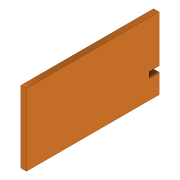
# Autodesk Inventor part: bottom_inner_wall
Saved by Autodesk Inventor 2020 (Build 240168000, 168)
## iProperties
Created: 2021-05-08
Part Number: bottom_inner_wall
Material: Gold
Document SubType Name: Modeling
Designer: Hsu Daniel
Density: 19.3 g/cm^3
Appearance: Metal 1600F Hot
Author: Hsu Daniel
Autodesk Inventor part; units mm, degrees
ref_plane "YZ Plane" through (0, 0, 0) normal (1, 0, 0) x (0, 1, 0)
ref_plane "XZ Plane" through (0, 0, 0) normal (0, 1, 0) x (-1, 0, 0)
ref_plane "XY Plane" through (0, 0, 0) normal (0, 0, 1) x (1, 0, 0)
sketch "Sketch1" plane through (0, 0, 0) normal (1, 0, 0) x (0, 1, 0)
  line L0 (0, 0) -> (71.7, 0)
  line L1 (71.7, 0) -> (71.7, -132.6)
  line L2 (71.7, -132.6) -> (0, -132.6)
  line L3 (0, -132.6) -> (0, 0)
  dimension "d0" = 71.7
  dimension "d1" = 132.6
  constraints: 8 end point, 2 parallel, 1 horizontal, 1 perpendicular
  measures "d0" distance of L1.end L2.end
  measures "d1" distance of L0.end L1.end
extrude "Extrusion1" add sketch "Sketch1" along normal blind 5.5
sketch "Sketch4" plane through (0, 0, 0) normal (-1, 0, 0) x (0, 0, 1)
  line L0 (-132.6, 0) -> (-132.6, 71.7) projected
  line L1 (-132.6, 25) -> (-122.6, 25)
  line L2 (-122.6, 25) -> (-122.6, 19.5)
  line L3 (-122.6, 19.5) -> (-132.6, 19.5)
  line L4 (-132.6, 19.5) -> (-132.6, 25)
  line L5 (0, 0) -> (-132.6, 0) projected
  dimension "d12" = 10
  dimension "d13" = 5.5
  dimension "d14" = 25
  constraints: 8 end point, 2 parallel, 1 horizontal, 1 perpendicular, 1 point on line
  measures "d12" distance of L2.end L3.end
  measures "d13" distance of L1.end L2.end
  measures "d14" distance between parallel lines of L5 L1
extrude "Extrusion4" cut sketch "Sketch4" against normal blind 5.5
sketch "Sketch2" plane through (5.5, 0, 0) normal (1, 0, 0) x (0, 0, -1)
  line L0 (119.2378, 76.9728) -> (81.7311, 76.9728)
  line L1 (81.7311, 76.9728) -> (81.7311, 64.0973)
  line L2 (81.7311, 64.0973) -> (119.2378, 64.0973)
  line L3 (119.2378, 64.0973) -> (119.2378, 76.9728)
  point P0 (0, 0)
  constraints: 8 end point, 2 parallel, 1 horizontal, 1 perpendicular
sketch "Sketch3" plane through (5.5, 0, 0) normal (1, 0, 0) x (0, 0, -1)
  line L0 (0, 71.7) -> (0, 0) projected
  line L1 (132.6, 0) -> (132.6, 71.7) projected
  line L2 (0, 0) -> (132.6, 0) projected
  line L3 (0, 19.5) -> (10, 19.5)
  line L4 (10, 19.5) -> (10, 25)
  line L5 (10, 25) -> (0, 25)
  line L6 (0, 25) -> (0, 19.5)
  point P0 (0, 50)
  dimension "d7" = 10
  dimension "d8" = 5.5
  dimension "d11" = 25
  constraints: 8 end point, 2 parallel, 1 horizontal, 1 perpendicular, 1 point on line
  measures "d7" distance of L5.end L4.end
  measures "d8" distance of L4.end L3.end
  measures "d11" distance between parallel lines of L2 L5
equation "\"d1\" = sidewallL"
equation "\"d14\" = wireH"
equation "\"d11\" = wireH"
equation "\"thick\" = 0.5"
equation "\"lrlr\" = 19"
equation "\"lrmid\" = 19.9"
equation "\"lrdepth\" = 3.3"
equation "\"mlr\" = 16.6"
equation "\"mmid\" = 24.7"
equation "\"mdepth\" = 4.5"
equation "\"lrltotal\" = 126.6"
equation "\"mltotal\" = 126.6"
equation "\"lrbetween\" = 52.1"
equation "\"mbetween\" = 49.5"
equation "\"toler\" = 1"
equation "\"tight\" = 0.08"
equation "\"stuckw\" = 6"
equation "\"sidewallL\" = 132.6"
equation "\"heaterH\" = 117.3"
equation "\"stickL\" = 3.5"
equation "\"wireH\" = 25"
body "Solid1"
